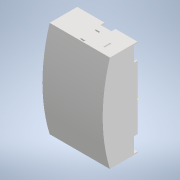
# Autodesk Inventor part: 3Dkrish
Saved by Autodesk Inventor 2022 (Build 260153000, 153)
## iProperties
Created: 2023-05-29
Part Number: 3Dkrish
Material: Типовые
Document SubType Name: Modeling
Designer: korsh624
Density: 1 g/cm^3
Appearance: По умолчанию
Author: korsh624
Autodesk Inventor part; units mm, degrees
ref_plane "YZ Plane" through (0, 0, 0) normal (1, 0, 0) x (0, 1, 0)
ref_plane "XZ Plane" through (0, 0, 0) normal (0, 1, 0) x (-1, 0, 0)
ref_plane "XY Plane" through (0, 0, 0) normal (0, 0, 1) x (1, 0, 0)
sketch "Эскиз1" plane through (0, 0, 0) normal (0, 0, 1) x (1, 0, 0)
  line L0 (-75.6484, -106.9824) -> (60.0028, -106.9824) projected
  line L1 (60.0028, 113.8664) -> (-75.6484, 113.8664) projected
  line L2 (-75.6484, -71.558) -> (-75.6484, 58.442) projected
  line L3 (60.0028, -71.558) -> (60.0028, 78.442) projected
  line L4 (63.0028, -109.9824) -> (-78.6484, -109.9824)
  line L5 (-78.6484, -109.9824) -> (-78.6484, 116.8664)
  line L6 (-78.6484, 116.8664) -> (63.0028, 116.8664)
  line L7 (63.0028, 116.8664) -> (63.0028, -109.9824)
  line L8 (60.0028, -106.9824) -> (-75.6484, -106.9824)
  line L9 (-75.6484, -106.9824) -> (-75.6484, 113.8664)
  line L10 (-75.6484, 113.8664) -> (60.0028, 113.8664)
  line L11 (60.0028, 113.8664) -> (60.0028, -106.9824)
  point P0 (0, 0)
  dimension "d0" = 3
  dimension "d1" = 3
  dimension "d2" = 3
  dimension "d3" = 3
  constraints: 16 end point, 4 parallel, 2 horizontal, 2 perpendicular
  measures "d0" distance between parallel lines of L4 L0
  measures "d1" distance between parallel lines of L1 L6
  measures "d2" distance between parallel lines of L2 L5
  measures "d3" distance between parallel lines of L7 L3
extrude "Выдавливание1" add sketch "Эскиз1" along normal blind 60
sketch "Эскиз2" plane through (63.0028, -109.9824, 0) normal (1, 0, 0) x (0, 0, -1)
  point P0 (0, 109.9824)
sketch "Эскиз3" plane through (0, 0, 0) normal (0, 0, -1) x (-1, 0, 0)
  point P0 (0, 0)
sketch "Эскиз4" plane through (63.0028, -109.9824, 0) normal (1, 0, 0) x (0, 0, -1)
  line L0 (-8, 38.4244) -> (-8, 3) projected
  line L1 (-8, 3) -> (-8, 38.4244) projected
  line L2 (0.0001, 223.8488) -> (0, 188.4244) projected
  line L3 (-8, 188.4244) -> (-7.9999, 223.8488) projected
  line L4 (0, 223.8488) -> (0, 3) projected
  line L5 (-8, 38.4244) -> (0, 38.4244)
  line L6 (0, 38.4244) -> (0, 3)
  line L7 (0, 3) -> (-8, 3)
  line L8 (-8, 3) -> (-8, 38.4244)
  line L9 (-7.9999, 223.8488) -> (0, 223.8488)
  line L10 (0, 223.8488) -> (0, 188.4244)
  line L11 (0, 188.4244) -> (-7.9999, 188.4244)
  line L12 (-7.9999, 188.4244) -> (-7.9999, 223.8488)
  point P0 (0, 109.9824)
  constraints: 16 end point, 4 parallel, 2 horizontal, 2 perpendicular
extrude "Выдавливание2" cut sketch "Эскиз4" against normal blind 239.25
sketch "Эскиз5" plane through (0, 0, 60) normal (0, 0, 1) x (1, 0, 0)
  line L0 (73.8028, -108.2777) -> (32.8028, -108.2777)
  line L1 (63.0028, 116.8664) -> (-78.6484, 116.8664) projected
  line L2 (-78.6484, 116.8664) -> (-78.6484, -109.9824) projected
  line L3 (-78.6484, -109.9824) -> (63.0028, -109.9824) projected
  line L4 (63.0028, -109.9824) -> (63.0028, 116.8664) projected
  line L5 (60.0028, 113.8664) -> (60.0028, -106.9824) projected
  line L6 (60.0028, -106.9824) -> (-75.6484, -106.9824) projected
  line L7 (-75.6484, -106.9824) -> (-75.6484, 113.8664) projected
  line L8 (-75.6484, 113.8664) -> (60.0028, 113.8664) projected
  line L9 (60.0028, -106.9824) -> (-75.6484, -106.9824) projected
  line L10 (-75.6484, 113.8664) -> (60.0028, 113.8664) projected
  line L11 (56.3016, -106.9824) -> (26.1407, -106.9824)
  line L12 (26.1407, -106.9824) -> (26.1407, 113.8664)
  line L13 (26.1407, 113.8664) -> (56.3016, 113.8664)
  line L14 (56.3016, 113.8664) -> (56.3016, -106.9824)
  line L15 (5.2877, -106.9824) -> (-25.8022, -106.9824)
  line L16 (-25.8022, -106.9824) -> (-25.8022, 113.8664)
  line L17 (-25.8022, 113.8664) -> (5.2877, 113.8664)
  line L18 (5.2877, 113.8664) -> (5.2877, -106.9824)
  line L19 (-48.9301, -106.9824) -> (-75.6484, -106.9824)
  line L20 (-75.6484, -106.9824) -> (-75.6484, 111.5008)
  line L21 (-75.6484, 111.5008) -> (-48.9301, 111.5008)
  line L22 (-48.9301, 111.5008) -> (-48.9301, -106.9824)
  line L23 (-75.6484, -106.9824) -> (-75.6484, 113.8664) projected
  line L24 (-75.6484, -32.9455) -> (-73.4662, -32.9455)
  line L25 (-73.4662, -32.9455) -> (-73.4662, -24.8216)
  line L26 (-73.4662, -24.8216) -> (-75.6484, -24.8216)
  line L27 (-75.6484, -24.8216) -> (-75.6484, -32.9455)
  line L28 (-75.6484, 29.4025) -> (-73.4662, 29.4025)
  line L29 (-73.4662, 29.4025) -> (-73.4662, 36.4767)
  line L30 (-73.4662, 36.4767) -> (-75.6484, 36.4767)
  line L31 (-75.6484, 36.4767) -> (-75.6484, 29.4025)
  point P0 (0, 0)
  constraints: 42 end point, 10 parallel, 9 point on line, 6 horizontal, 5 perpendicular, 2 other
extrude "Выдавливание3" add sketch "Эскиз5" along normal blind 5 contours L4 L3 L2 L1 | L14 L6 L12 L8 | L18 L6 L16 L8 | L6 L7 L24 L25 L26 L28 L29 L30 L21 L22
sketch "Эскиз6" plane through (0, 0, 65) normal (0, 0, 1) x (1, 0, 0)
  line L0 (-48.9301, 111.5008) -> (-75.6484, 111.5008) projected
  line L1 (-75.6484, 111.5008) -> (-75.6484, 113.8664) projected
  line L2 (-48.9301, 111.5008) -> (-75.6484, 111.5008)
  line L3 (-75.6484, 111.5008) -> (-75.6484, 113.8664)
  line L4 (-75.6484, 113.8664) -> (-48.9301, 113.8664)
  line L5 (-48.9301, 113.8664) -> (-48.9301, 111.5008)
  point P0 (0, 0)
  constraints: 8 end point, 2 parallel, 1 horizontal, 1 perpendicular
extrude "Выдавливание4" add sketch "Эскиз6" against normal blind 5
sketch "Эскиз7" plane through (-78.6484, -71.558, 0) normal (-1, 0, 0) x (0, 0, 1)
  point P0 (0, 71.558)
sketch "Эскиз8" plane through (-78.6484, 116.8664, 0) normal (0, 1, 0) x (1, 0, 0)
  line L0 (85.4799, -9.5) -> (62.4799, -9.5) projected
  line L1 (74.1362, -4.2225) -> (79.8964, -4.2225) projected
  line L2 (141.6512, 0) -> (0, 0) projected
  line L3 (85.4799, -9.5) -> (64.1362, -9.5)
  line L4 (64.1362, -9.5) -> (64.1362, 0)
  line L5 (64.1362, 0) -> (85.4799, 0)
  line L6 (85.4799, 0) -> (85.4799, -9.5)
  line L7 (64.1362, -9.5) -> (89.8964, -9.5)
  line L8 (89.8964, -9.5) -> (89.8964, 0)
  line L9 (89.8964, 0) -> (64.1362, 0)
  line L10 (64.1362, 0) -> (64.1362, -9.5)
  point P0 (78.6484, 0)
  dimension "d12" = 10
  dimension "d13" = 5.584
  dimension "d14" = 10
  constraints: 16 end point, 4 parallel, 2 horizontal, 2 perpendicular, 2 point on line
  measures "d12" distance from line of L4 L1.start
  measures "d14" distance from line of L8 L1.end
extrude "Выдавливание5" cut sketch "Эскиз8" against normal blind 5
sketch "Эскиз9" plane through (63.0028, -71.558, 0) normal (1, 0, 0) x (0, 0, -1)
  line L0 (-65, -38.4244) -> (-65, 188.4244) projected
  arc A0 (-65, 188.4244) -> (-65, -38.4244) centre (307.5062, 75) ccw
  line L1 (0, -38.4244) -> (-65, -38.4244) projected
  line L2 (-65, -38.4244) -> (-65, -28.4244)
  line L3 (-65, -28.4244) -> (-65, 178.4244)
  arc A1 (-65, 178.4244) -> (-65, -28.4244) centre (307.5062, 75) ccw
  point P0 (0, 71.558)
  dimension "d17" = 10
  dimension "d18" = 10
  constraints: 4 end point, 4 point on circle, 2 centre point, 2 point on line
  measures "d17" distance of L0.start L2.end
  measures "d18" distance of L3.end L0.end
extrude "Выдавливание6" add sketch "Эскиз9" against normal blind 141.651 contours A0 L0 A1
sketch "Эскиз10" plane through (63.0028, -71.558, 0) normal (1, 0, 0) x (0, 0, -1)
  arc A0 (-65, 178.4244) -> (-65, -28.4244) centre (307.5062, 75) ccw projected
  line L0 (-65, -28.4244) -> (-65, 178.4244) projected
  point P0 (0, 71.558)
extrude "Выдавливание7" add sketch "Эскиз10" against normal blind 3
sketch "Эскиз11" plane through (-78.6484, -71.558, 0) normal (-1, 0, 0) x (0, 0, 1)
  arc A0 (65, -28.4244) -> (65, 178.4244) centre (-307.5062, 75) ccw projected
  line L0 (65, 188.4244) -> (65, -38.4244) projected
  point P0 (0, 71.558)
extrude "Выдавливание8" add sketch "Эскиз11" against normal blind 3
sketch "Эскиз12" plane through (-78.6484, -109.9824, 0) normal (0, -1, 0) x (1, 0, 0)
  spline S0 degree 3 poles (75.9334, 40.3738) (75.8831, 40.8501) (75.7622, 41.3112) (75.3324, 42.3118) (75.0359, 42.7084) (74.4654, 43.3771) (73.9913, 43.782) (72.8589, 44.371) (72.2642, 44.5465) (71.3446, 44.633) (71.0335, 44.6318) (70.0476, 44.5299) (69.4546, 44.3267) (68.4476, 43.7801) (67.9673, 43.407) (67.0987, 42.3576) (66.8298, 41.785) (66.5793, 40.9818) (66.515, 40.667) (66.4421, 39.9332) (66.4622, 39.6005) (66.486, 39.3756) knots -0.649055 -0.649055 -0.649055 -0.649055 -0.611574 -0.611574 -0.563504 -0.563504 -0.482019 -0.482019 -0.407033 -0.407033 -0.368981 -0.368981 -0.286973 -0.286973 -0.207347 -0.207347 -0.121004 -0.121004 -0.067856 -0.067856 0 0 0 0 projected
  spline S1 degree 3 poles (66.486, 39.3756) (66.5097, 39.1507) (66.5596, 38.8211) (66.7843, 38.1188) (66.913, 37.8244) (67.3257, 37.0912) (67.7084, 36.5875) (68.7772, 35.7428) (69.3247, 35.4783) (70.4238, 35.1543) (71.0461, 35.0795) (72.0316, 35.1858) (72.3361, 35.2497) (73.2173, 35.5265) (73.7622, 35.8224) (74.7465, 36.635) (75.1255, 37.13) (75.5436, 37.9033) (75.7507, 38.353) (75.9619, 39.4214) (75.9837, 39.8976) (75.9334, 40.3738) knots -2.488 -2.488 -2.488 -2.488 -2.22789 -2.22789 -2.024159 -2.024159 -1.693184 -1.693184 -1.387958 -1.387958 -1.073596 -1.073596 -0.927734 -0.927734 -0.640291 -0.640291 -0.327938 -0.327938 -0.143673 -0.143673 0 0 0 0 projected
  point P0 (78.6484, 0)
extrude "Выдавливание9" cut sketch "Эскиз12" against normal blind 3
sketch "Эскиз13" plane through (-78.6484, 116.8664, 65) normal (0, 1, 0) x (1, 0, 0)
  line L0 (49.8619, 5.8292) -> (89.8619, 5.8292) projected
  line L1 (89.8619, 37.7292) -> (49.8619, 37.7292) projected
  line L2 (101.9119, 18.2982) -> (101.9119, 14.2982) projected
  line L3 (101.9119, 29.2602) -> (101.9119, 25.2602) projected
  line L4 (77.7841, 5.8292) -> (67.7841, 5.8292)
  line L5 (67.7841, 5.8292) -> (67.7841, 2.8292)
  line L6 (67.7841, 2.8292) -> (77.7841, 2.8292)
  line L7 (77.7841, 2.8292) -> (77.7841, 5.8292)
  line L8 (77.7841, 37.7292) -> (67.7841, 37.7292)
  line L9 (67.7841, 37.7292) -> (67.7841, 40.7292)
  line L10 (67.7841, 40.7292) -> (77.7841, 40.7292)
  line L11 (77.7841, 40.7292) -> (77.7841, 37.7292)
  line L12 (111.7909, 14.2982) -> (114.7909, 14.2982)
  line L13 (114.7909, 14.2982) -> (114.7909, 29.2602)
  line L14 (114.7909, 29.2602) -> (111.7909, 29.2602)
  line L15 (111.7909, 29.2602) -> (111.7909, 14.2982)
  point P0 (78.6484, 65)
  point P1 (67.7841, 5.8292)
  dimension "d27" = 10
  dimension "d28" = 3
  dimension "d29" = 3
  dimension "d30" = 3
  constraints: 24 end point, 6 parallel, 4 point on line, 3 horizontal, 3 perpendicular
  measures "d27" distance of L6.end L5.end
  measures "d28" distance of L5.end L4.end
  measures "d29" distance of L8.end L9.end
  measures "d30" distance of L14.end L13.end
extrude "Выдавливание10" cut sketch "Эскиз13" against normal blind 3
sketch "Эскиз14" plane through (-78.6484, 116.8664, 65) normal (0, 1, 0) x (1, 0, 0)
  circle A0 centre (26.4286, 24.6652) radius 8
  point P0 (78.6484, 65)
  dimension "d33" = 16
  constraints: 1 centre point
  measures "d33" diameter of A0
extrude "Выдавливание11" cut sketch "Эскиз14" against normal blind 3
chamfer "Фаска1" distance 2 angle 45 1 edges at (-60.2198, 116.8664, 40.3348)
sketch "Эскиз15" plane through (-78.6484, -71.558, 0) normal (-1, 0, 0) x (0, 0, 1)
  line L0 (-6, 73) -> (-6, 77) projected
  line L1 (-6, 73) -> (-6, 77) projected
  circle A0 centre (10, 75) radius 1.5
  line L2 (0, 150) -> (0, 0) projected
  point P0 (0, 71.558)
  dimension "d39" = 3
  dimension "d40" = 10
  constraints: 1 centre point
  measures "d39" diameter of A0
  measures "d40" distance from line of A0.centre L2
extrude "Выдавливание12" cut sketch "Эскиз15" against normal blind 560
sketch "Эскиз16" plane through (0, 0, 0) normal (0, 0, -1) x (-1, 0, 0)
  line L0 (75.6484, -71.558) -> (78.6484, -71.558) projected
  line L1 (78.6484, 78.442) -> (78.6484, -71.558) projected
  line L2 (78.6484, 78.442) -> (75.6484, 78.442) projected
  line L3 (75.6484, -71.558) -> (75.6484, 78.442) projected
  line L4 (-63.0028, -71.558) -> (-60.0028, -71.558) projected
  line L5 (-60.0028, 78.442) -> (-60.0028, -71.558) projected
  line L6 (-60.0028, 78.442) -> (-63.0028, 78.442) projected
  line L7 (-63.0028, -71.558) -> (-63.0028, 78.442) projected
  line L8 (78.6484, -106.9824) -> (-63.0028, -106.9824) projected
  line L9 (-63.0028, -109.9824) -> (-63.0028, -106.9824) projected
  line L10 (78.6484, -109.9824) -> (-63.0028, -109.9824) projected
  line L11 (78.6484, -106.9824) -> (78.6484, -109.9824) projected
  line L12 (-11.248, 113.8664) -> (-11.248, 116.8664) projected
  line L13 (-63.0028, 116.8664) -> (-11.248, 116.8664) projected
  line L14 (-63.0028, 113.8664) -> (-63.0028, 116.8664) projected
  line L15 (-63.0028, 113.8664) -> (-11.248, 113.8664) projected
  line L16 (14.5122, 116.8664) -> (14.5122, 113.8664) projected
  line L17 (14.5122, 113.8664) -> (78.6484, 113.8664) projected
  line L18 (78.6484, 116.8664) -> (78.6484, 113.8664) projected
  line L19 (14.5122, 116.8664) -> (78.6484, 116.8664) projected
  point P0 (0, 0)
extrude "Выдавливание13" add sketch "Эскиз16" along normal blind 6
equation "\"d2\" = d1"
equation "\"d3\" = d0"
